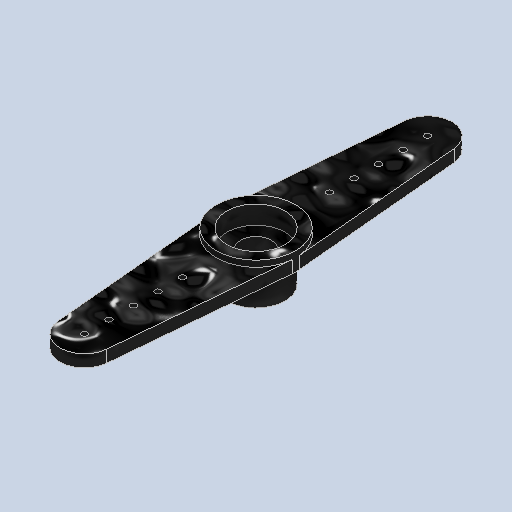
# Autodesk Inventor part: ServoMotor_Hone1
Saved by Autodesk Inventor 2022 (Build 260153000, 153)
## iProperties
Created: 2024-09-23
Part Number: ServoMotor_Hone1
Material: 一般
Document SubType Name: Modeling
Designer: acbaf
Density: 1 g/cm^3
Appearance: 黒
Author: acbaf
Autodesk Inventor part; units mm, degrees
ref_plane "YZ Plane" through (0, 0, 0) normal (1, 0, 0) x (0, 1, 0)
ref_plane "XZ Plane" through (0, 0, 0) normal (0, 1, 0) x (-1, 0, 0)
ref_plane "XY Plane" through (0, 0, 0) normal (0, 0, 1) x (1, 0, 0)
sketch "スケッチ1" plane through (0, 0, 0) normal (0, 1, 0) x (-1, 0, 0)
  circle A0 centre (0, 0) radius 2.5
  circle A1 centre (0, 0) radius 4.75
  line L0 (0, 0) -> (0, -28)
  line L1 (0, 0) -> (0, 28)
  circle A2 centre (0, 0) radius 6.5
  circle A3 centre (0, 28) radius 4
  line L2 (6.5, 0) -> (-6.5, 0)
  circle A4 centre (0, -28) radius 4
  line L3 (6.474, 0.5804) -> (3.984, 28.3571)
  line L4 (-3.984, 28.3571) -> (-6.474, 0.5804)
  line L5 (-6.474, -0.5804) -> (-3.984, -28.3571)
  line L6 (6.474, -0.5804) -> (3.984, -28.3571)
  circle A5 centre (0, -28) radius 0.5
  circle A6 centre (0, -24) radius 0.5
  circle A7 centre (0, -20) radius 0.5
  circle A8 centre (0, -16) radius 0.5
  circle A9 centre (0, -12) radius 0.5
  circle A10 centre (0, 28) radius 0.5
  circle A11 centre (0, 24) radius 0.5
  circle A12 centre (0, 20) radius 0.5
  circle A13 centre (0, 16) radius 0.5
  circle A14 centre (0, 12) radius 0.5
  dimension "d0" = 5
  dimension "d1" = 9.5
  dimension "d2" = 28
  dimension "d3" = 28
  dimension "d4" = 13
  dimension "d5" = 8
  dimension "d6" = 0
  dimension "d7" = 0
  dimension "d8" = 1
  dimension "d9" = 1
  dimension "d10" = 4
  dimension "d11" = 1
  dimension "d12" = 1
  dimension "d13" = 1
  dimension "d14" = 4
  dimension "d15" = 4
  dimension "d16" = 4
  constraints: 15 centre point, 14 end point, 10 point on circle, 8 tangent, 6 symmetric about line, 5 coincident, 4 point on line, 2 vertical, 6 other
  measures "d0" diameter of A0
  measures "d1" diameter of A1
  measures "d2" distance of L0.start L0.end
  measures "d3" distance of L0.start L1.end
  measures "d4" diameter of A2
  measures "d5" diameter of A3
  measures "d6" distance from line of L0 A4.centre
  measures "d7" distance from line of L2 A0.centre
  measures "d8" diameter of A5
  measures "d9" diameter of A6
  measures "d10" distance of L0.end A6.centre
  measures "d11" diameter of A7
  measures "d12" diameter of A8
  measures "d13" diameter of A9
  measures "d14" distance of A6.centre A7.centre
  measures "d15" distance of A7.centre A8.centre
  measures "d16" distance of A9.centre A8.centre
extrude "押し出し1" add sketch "スケッチ1" along normal blind 2 contours A2 L4 A3 A11 L1 A12 A13 A14 | L1 A14 A13 A12 A11 A3 L3 A2 | A2 L6 A4 A6 L0 A7 A8 A9 | L0 A9 A8 A7 A6 A4 L5 A2 | A3 A11 | A4 A6
extrude "押し出し2" add sketch "スケッチ1" along normal blind 3 contours L2 A2 L0 A1 | A1 L1 A2 L2 | A1 L2 A2 L1 | L0 A2 L2 A1
extrude "押し出し3" add sketch "スケッチ1" against normal blind 5 contours L2 A1 L0 A0 | A0 L1 A1 L2 | A0 L2 A1 L1 | L0 A1 L2 A0
equation "\"d14\" = d10"
equation "\"d15\" = d14"
equation "\"d16\" = d15"
